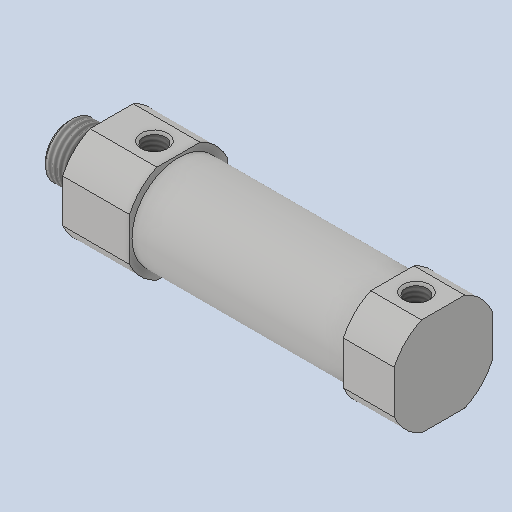
# Autodesk Inventor part: CJ2B16-15Z-B(1_0)_BODY
Saved by Autodesk Inventor 2025.1 (Build 291241000, 241)
## iProperties
Created: 2024-03-16
Part Number: CJ2B16-15Z-B(1_0)_BODY
Material: Generic
Catalog Web Link: www.cadenas.de
Description: CJ2-Z BODY-Air Cylinder/Standard: Double Acting Single Rod
Vendor: SMC
Document SubType Name: Modeling
Designer: psAdmin
Manufacturer: SMC
Mass: 12.0684 g
Surface Area: 63.1293 cm^2
Volume: 12.0684 cm^3
Density: 1 g/cm^3
Appearance: PSOLRGB-175-175-175
Category: PARTsolutions
Company: SMC
PSOL_IDENT_0: {$CADENAS_DATA/23d-libs/smc_jp/actuator/standard_air_cylinder/cj2/cj2_z/parts/cj2_z_body.prj},265 {V
PSOL_IDENT_1: TYP=3D},{NB=CJ2B16-15Z-B(1_0)_BODY},{LINA=CJ2B16-15Z-B_BODY},{NN=CJ2-Z BODY},{DATE=07.03.2024 03:01:
PSOL_IDENT_2: 52},{GEOMDATE=28.10.2023 01:41:00},{VERSION=},{LINEID=410},{WBVAR=AUTOSWITCH,NUMBER,CUSHION,STOP,STR
PSOL_IDENT_3: OKE,PORT,MOUNTING,OMSCXC3,OMSCXC51,THREAD},{WBNUMERIC=STROKE}  {NB=CJ2B16-15Z-B(1_0)_BODY},{LINA=CJ2
PSOL_IDENT_4: B16-15Z-B_BODY},{KT=DUMMY},{ORDER=CJ2B16-15Z-B},{BORE=16},{MOUNT=(B) Basic},{AUTOSWITCH=},{NUMBER=},
PSOL_IDENT_5: {CUSHION=},{MOUNTX=B},{STOP=1},{STROKE=15},{SMAX=400},{PORT=},{MOUNTING=-B},{OMSCXC3=},{OMSCXC51=},{
PSOL_IDENT_6: THREAD=0},{B=18.3},{B1X1=18.3},{B2=18.300},{C=20},{C1X1=20.0},{C2=20.000},{CD=0.0},{U=0},{CX=0.0},{C
PSOL_IDENT_7: Z=0},{CZ1X1=0.0},{D=5},{F=8},{GA=8.0},{GA1X1=8.0},{GA2=7.500},{GB=5.0},{GB1X1=5.0},{GB2=6.500},{H=28
PSOL_IDENT_8: },{NA=12.5},{NA1X1=12.5},{NA2=21.000},{NB1=9.5},{NB1X1=9.5},{NB2=20.000},{NDH8=10 0/-0.022},{NDH81=1
PSOL_IDENT_9: 0},{NN=M10x1.0},{NN1=10},{NN2=1.0},{R=0},{S=47},{S1X1=47.0},{S2X2=66.000},{WA=14.5},{WB=13.5},{WW=5.
PSOL_IDENT_10: 5},{MOUNTINGX='','(-) None','-A','(A) Rail mounting','-B','(B) Band mounting'},{PORTX='', '(-) Perpe
PSOL_IDENT_11: ndicular', 'R', '(R) In-line'},{SWX=6.5},{SW1=6.500},{SW2=2.500},{SW3=3.000},{SW4=2.000},{SW5=5.000}
PSOL_IDENT_12: ,{SW6=1.000},{SW7=3.500},{SW8=4.000},{SW9=1.000},{SW=6.5},{SWSINX= '','N/A' },{NENN=CJ2B16},{X1=6.00
PSOL_IDENT_13: 0},{X2=7.500},{Y1=3.000},{Y2=6.500},{X=6},{Y=3},{XC3= '','(-) None','-XC3AB','(XC3AB) Rod port locat
PSOL_IDENT_14: ion viewed: A,Head port location viewed: B','-XC3AC','(XC3AC) Rod port location viewed: A,Head port
PSOL_IDENT_15: location viewed: C','-XC3AD','(XC3AD) Rod port location viewed: A,Head port location viewed: D','-XC
PSOL_IDENT_16: 3BA','(XC3BA) Rod port location viewed: B,Head port location viewed: A','-XC3BB','(XC3BB) Rod port l
PSOL_IDENT_17: ocation viewed: B,Head port location viewed: B','-XC3BC','(XC3BC) Rod port location viewed: B,Head p
PSOL_IDENT_18: ort location viewed: C','-XC3BD','(XC3BD) Rod port location viewed: B,Head port location viewed:D','
PSOL_IDENT_19: -XC3CA','(XC3CA) Rod port location viewed: C,Head port location viewed: A','-XC3CB','(XC3CB) Rod por
PSOL_IDENT_20: t location viewed: C,Head port location viewed: B','-XC3CC','(XC3CC) Rod port location viewed: C,Hea
PSOL_IDENT_21: d port location viewed: C','-XC3CD','(XC3CD) Rod port location viewed: C,Head port location viewed:D'
PSOL_IDENT_22: ,'-XC3DA','(XC3DA) Rod port location viewed: D,Head port location viewed: A','-XC3DB','(XC3DB) Rod p
PSOL_IDENT_23: ort location viewed: D,Head port location viewed: B','-XC3DC','(XC3DC) Rod port location viewed: D,H
PSOL_IDENT_24: ead port location viewed: C','-XC3DD','(XC3DD) Rod port location viewed: D,Head port location viewed
PSOL_IDENT_25: :D' },{PORTXC3=A1},{PORTXC32=A2},{CUSHIONX= '','(-) Rubber cushion','A','(A) Air cushion' },{XC51= ''
PSOL_IDENT_26: ,'(-) None','-XC51H4','(XC51H4) Hose nipple type: ø4/2.5 with restriction','-XC51H6','(XC51H6) Hose
PSOL_IDENT_27: nipple type: ø6/4 with restriction','-XC51MH4','(XC51MH4) Hose nipple type: ø4/2.5 without restricti
PSOL_IDENT_28: on','-XC51MH6','(XC51MH6) Hose nipple type: ø6/4 without restriction' },{MODEL=M-5H-6},{PINMODEL=CD-
PSOL_IDENT_29: Z015}
NB: CJ2B16-15Z-B(1_0)_BODY
NN: M10x1.0
NT: Air Cylinder/Standard: Double Acting Single Rod
NBSYN: $ORDER.($STOP._$THREAD.)_BODY
LINA: CJ2B16-15Z-B_BODY
CATALOG: SMC (JP
ROWDESC: CJ2B16
BORE: 16
MOUNT: (B) Basic
AUTOSWITCH: (-) Without autoswitch
NUMBER: N/A
CUSHION: (-) Rubber cushion
STOP: Manufacturable stroke
STROKE: 15
SMAX: 400
PORT: (-) Perpendicular
MOUNTING: (B) Band mounting
OMSCXC3: (-) None
OMSCXC51: (-) None
THREAD: on
B: 18.3
B1X1: 18.3
B2: 18.3
C: 20
C1X1: 20
C2: 20
CD: 0
U: 0
CX: 0
CZ: 0
CZ1X1: 0
D: 5
F: 8
GA: 8
GA1X1: 8
GA2: 7.5
GB: 5
GB1X1: 5
GB2: 6.5
H: 28
NA: 12.5
NA1X1: 12.5
NA2: 21
NB1: 9.5
NB1X1: 9.5
NB2: 20
NDH8: 10 0/-0.022
NDH81: 10
NN1: 10
NN2: 1
R: 0
S: 47
S1X1: 47
S2X2: 66
WA: 14.5
WB: 13.5
WW: 5.5
SW1: 6.5
SW2: 2.5
SW3: 3
SW4: 2
SW5: 5
SW6: 1
SW7: 3.5
SW8: 4
SW9: 1
X1: 6
X2: 7.5
Y1: 3
Y2: 6.5
SUPPLIER: SMC
ARTICLENO: CJ2B16-15Z-B(1_0)_BODY
BOMINFO: CJ2B16-15Z-B_BODY
CREATOR: CADENAS GmbH
Title: CJ2B16-15Z-B_BODY
Author: Cadenas PARTsolutions
Comments: Air Cylinder/Standard: Double Acting Single Rod
Autodesk Inventor part; units mm, degrees
sketch "Sketch_8" plane through (0, 0, 0) normal (0, 0, 1) x (1, 0, 0)
  line L0 (0, 0) -> (-8, 0)
  line L1 (-8, 0) -> (-8, 4.3865)
  line L2 (-8, 4.3865) -> (-7.3865, 5)
  line L3 (-7.3865, 5) -> (0, 5)
  line L4 (0, 5) -> (0, 0)
  line L5 (0, 0) -> (-8, 0)
  constraints: 12 end point
revolve "Revolution1" add sketch "Sketch_8" angle 360 about axis through (0, 0, 0) along (1, 0, 0)
thread "Thread1" size "M10x1" class "6g" standard "ISO Metric profile" length 5.8865
sketch "Sketch_9" plane through (0, 0, 0) normal (1, 0, 0) x (0, 0, -1)
  line L0 (-9.15, 4.0345) -> (-9.15, -4.0345)
  arc A0 (-9.15, -4.0345) -> (-4.0345, -9.15) centre (0, 0) ccw
  line L1 (-4.0345, -9.15) -> (4.0345, -9.15)
  arc A1 (4.0345, -9.15) -> (9.15, -4.0345) centre (0, 0) ccw
  line L2 (9.15, -4.0345) -> (9.15, 4.0345)
  arc A2 (9.15, 4.0345) -> (4.0345, 9.15) centre (0, 0) ccw
  line L3 (4.0345, 9.15) -> (-4.0345, 9.15)
  arc A3 (-4.0345, 9.15) -> (-9.15, 4.0345) centre (0, 0) ccw
  constraints: 8 end point, 8 point on circle, 4 centre point
extrude "Extrusion1" add sketch "Sketch_9" along normal blind 12.5
sketch "Sketch_11" plane through (12.5, 0, 0) normal (1, 0, 0) x (0, 0, -1)
  circle A0 centre (0, 0) radius 8.7
  constraints: 1 centre point
extrude "Extrusion2" add sketch "Sketch_11" along normal blind 40
sketch "Sketch_10" plane through (52.5, 0, 0) normal (1, 0, 0) x (0, 0, -1)
  line L0 (-9.15, 4.0345) -> (-9.15, -4.0345)
  arc A0 (-9.15, -4.0345) -> (-4.0345, -9.15) centre (0, 0) ccw
  line L1 (-4.0345, -9.15) -> (4.0345, -9.15)
  arc A1 (4.0345, -9.15) -> (9.15, -4.0345) centre (0, 0) ccw
  line L2 (9.15, -4.0345) -> (9.15, 4.0345)
  arc A2 (9.15, 4.0345) -> (4.0345, 9.15) centre (0, 0) ccw
  line L3 (4.0345, 9.15) -> (-4.0345, 9.15)
  arc A3 (-4.0345, 9.15) -> (-9.15, 4.0345) centre (0, 0) ccw
  constraints: 8 end point, 8 point on circle, 4 centre point
extrude "Extrusion3" add sketch "Sketch_10" along normal blind 9.5
sketch "Sketch5" plane through (0, 9.15, 4.0345) normal (0, 1, 0) x (1, 0, 0)
  point P0 (8, 4.0345)
hole "Hole1" at (8, 9.15, 0) direction (0, -1, 0) diameter 4.134 depth 5 tip angle 120 countersink diameter 5 countersink angle 90 thread size "M5x0.8" class "6H" standard "ISO Metric profile"
sketch "Sketch6" plane through (52.5, 9.15, 4.0345) normal (0, 1, 0) x (1, 0, 0)
  point P0 (4.5, 4.0345)
hole "Hole2" at (57, 9.15, 0) direction (0, -1, 0) diameter 4.134 depth 5 tip angle 120 countersink diameter 5 countersink angle 90 thread size "M5x0.8" class "6H" standard "ISO Metric profile"
sketch "Sketch_16" plane through (0, 0, 0) normal (0, 0, 1) x (1, 0, 0)
  line L0 (32.5, 0) -> (-8, 0)
  line L1 (-8, 0) -> (-8, 2.5)
  line L2 (-8, 2.5) -> (12.5, 2.5)
  line L3 (12.5, 2.5) -> (12.5, 8)
  line L4 (12.5, 8) -> (32.5, 8)
  line L5 (32.5, 8) -> (32.5, 0)
  line L6 (32.5, 0) -> (-8, 0)
  constraints: 14 end point
revolve "Revolution2" cut sketch "Sketch_16" angle 360 about axis through (32.5, 0, 0) along (1, 0, 0)
ref_plane "BODY_N_XY" through (62, 0, 0) normal (0, 0, -1) x (1, 0, 0)
ref_plane "BODY_N_YZ" through (62, 0, 0) normal (1, 0, 0) x (0, -1, 0)
ref_plane "BODY_N_ZX" through (62, 0, 0) normal (0, -1, 0) x (0, 0, -1)
ref_plane "NUT2_XY" through (62, 0, 0) normal (1, 0, 0) x (0, 0, -1)
ref_plane "NUT2_YZ" through (62, 0, 0) normal (0, 0, -1) x (0, 1, 0)
ref_plane "NUT2_ZX" through (62, 0, 0) normal (0, 1, 0) x (1, 0, 0)
ref_plane "SW1_XY" through (19, 0, 0) normal (1, 0, 0) x (0, 0, -1)
ref_plane "SW1_YZ" through (19, 0, 0) normal (0, 0, -1) x (0, 1, 0)
ref_plane "SW1_ZX" through (19, 0, 0) normal (0, 1, 0) x (1, 0, 0)
ref_plane "SW2_XY" through (46, 0, 0) normal (-1, 0, 0) x (0, 0, -1)
ref_plane "SW2_YZ" through (46, 0, 0) normal (0, 0, -1) x (0, -1, 0)
ref_plane "SW2_ZX" through (46, 0, 0) normal (0, -1, 0) x (-1, 0, 0)
ref_plane "SW_R1_XY" through (19, -14.15, 0) normal (1, 0, 0) x (0, 0, -1)
ref_plane "SW_R1_YZ" through (19, -14.15, 0) normal (0, 0, -1) x (0, 1, 0)
ref_plane "SW_R1_ZX" through (19, -14.15, 0) normal (0, 1, 0) x (1, 0, 0)
ref_plane "SW_R2_XY" through (46, -14.15, 0) normal (-1, 0, 0) x (0, 0, -1)
ref_plane "SW_R2_YZ" through (46, -14.15, 0) normal (0, 0, -1) x (0, -1, 0)
ref_plane "SW_R2_ZX" through (46, -14.15, 0) normal (0, -1, 0) x (-1, 0, 0)
ref_plane "body_XY" through (0, 0, 0) normal (-1, 0, 0) x (0, 0, -1)
ref_plane "body_YZ" through (0, 0, 0) normal (0, 0, -1) x (0, -1, 0)
ref_plane "body_ZX" through (0, 0, 0) normal (0, -1, 0) x (-1, 0, 0)
body "Solid1"
